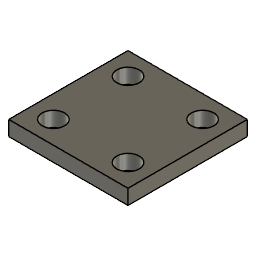
BoTech.StarClock.Connector (Autodesk Fusion 360 design; units mm, degrees)
Autodesk Fusion 360 part; units mm, degrees
sketch "Skizze1" plane through (0, 0, 0) normal (0, 0, 1) x (1, 0, 0)
  line L0 (5, -5) -> (-5, -5)
  circle A0 centre (-5, -5) radius 1.5
  line L1 (-5, -5) -> (-5, 5)
  circle A1 centre (-5, 5) radius 1.5
  line L2 (5, 5) -> (5, -5)
  line L3 (-5, 5) -> (5, 5)
  circle A2 centre (5, 5) radius 1.5
  circle A3 centre (5, -5) radius 1.5
  line L4 (-8, 8) -> (8, 8)
  line L5 (8, 8) -> (8, -8)
  line L6 (8, -8) -> (-8, -8)
  line L7 (-8, -8) -> (-8, 8)
  dimension "d1" = 10
  dimension "d2" = 10
  dimension "d3" = 3
  dimension "d4" = 3
  dimension "d5" = 3
  dimension "d6" = 3
  dimension "d7" = 16
  dimension "d8" = 16
  constraint horizontal L0
  constraint vertical L1
  constraint horizontal L3
  constraint vertical L2
  constraint coincident L0.start L2.end
  constraint coincident L0.end A0.centre
  constraint coincident L2.start L3.end
  constraint coincident L1.end A1.centre
  constraint horizontal L4
  constraint vertical L5
  constraint horizontal L6
  constraint vertical L7
  measures "d1" distance of L0.start L0.end
  measures "d2" distance of L0.start L2.start
  measures "d3" diameter of A3
  measures "d4" diameter of A0
  measures "d5" diameter of A2
  measures "d6" diameter of A1
  measures "d7" distance of L4.start L4.end
  measures "d8" distance of L4.start L6.end
extrude "Extrusion1" add sketch "Skizze1" along normal blind 2 contours L0 A0 L1 A1 L2 L3 A2 A3 | L4 L5 L6 L7
